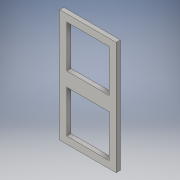
# Autodesk Inventor part: ClawExtender
Saved by Autodesk Inventor 2016 (Build 200138000, 138)
## iProperties
Created: 2016-04-28
Part Number: ClawExtender
Material: Generic
Document SubType Name: Modeling
Designer: mkepler
Density: 1 g/cm^3
Appearance: Default
Author: mkepler
Autodesk Inventor part; units mm, degrees
ref_plane "YZ Plane" through (0, 0, 0) normal (1, 0, 0) x (0, 1, 0)
ref_plane "XZ Plane" through (0, 0, 0) normal (0, 1, 0) x (-1, 0, 0)
ref_plane "XY Plane" through (0, 0, 0) normal (0, 0, 1) x (1, 0, 0)
sketch "Sketch1" plane through (0, 0, 0) normal (0, 1, 0) x (-1, 0, 0)
  line L0 (0, 0) -> (40, 0)
  line L1 (40, 0) -> (40, -80)
  line L2 (40, -80) -> (0, -80)
  line L3 (0, -80) -> (0, 0)
  dimension "d0" = 40
  dimension "d1" = 80
  constraints: 8 end point, 2 perpendicular, 1 horizontal, 1 vertical
  measures "d0" distance of L0.start L0.end
  measures "d1" distance of L0.end L1.end
extrude "Extrusion1" add sketch "Sketch1" along normal blind 3
sketch "Sketch3" plane through (0, 3, 0) normal (0, 1, 0) x (1, 0, 0)
  line L0 (-40, 0) -> (0, 0) projected
  line L1 (-40, 0) -> (-40, 5)
  line L2 (-35, 5) -> (-5, 5)
  line L3 (0, 5) -> (0, 35)
  line L4 (0, 0) -> (0, 80) projected
  line L5 (-5, 35) -> (-35, 35)
  line L6 (-40, 80) -> (-40, 0) projected
  line L7 (-40, 35) -> (-40, 45)
  line L8 (0, 45) -> (-35, 45)
  line L9 (0, 45) -> (0, 75)
  line L10 (-5, 75) -> (-35, 75)
  line L11 (0, 80) -> (-40, 80) projected
  line L12 (-40, 80) -> (-35, 80)
  line L13 (0, 80) -> (-5, 80)
  line L14 (-5, 75) -> (-5, 45)
  line L15 (-5, 35) -> (-5, 5)
  line L16 (-35, 75) -> (-35, 45)
  line L17 (-35, 35) -> (-35, 5)
  dimension "d4" = 5
  dimension "d5" = 30
  dimension "d6" = 10
  dimension "d7" = 30
  dimension "d8" = 5
  dimension "d9" = 5
  constraints: 28 end point, 8 point on line, 7 perpendicular, 1 parallel, 1 vertical
  measures "d4" distance of L0.start L1.end
  measures "d5" distance of L3.start L3.end
  measures "d6" distance of L7.start L7.end
  measures "d7" distance of L8.start L9.end
  measures "d8" distance of L6.start L12.end
  measures "d9" distance of L4.end L13.end
extrude "Extrusion2" cut sketch "Sketch3" against normal through all contours L8 L16 L10 L14 | L17 L5 L15 L2
body "Solid1"
